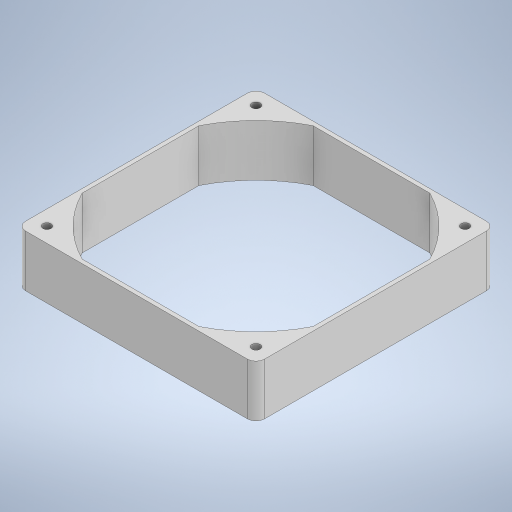
# Autodesk Inventor part: 120mm_fan
Saved by Autodesk Inventor 2023 (Build 270158000, 158)
## iProperties
Created: 2023-08-19
Part Number: 120mm_fan
Material: Generic
Document SubType Name: Modeling
Designer: plebbb
Density: 1 g/cm^3
Appearance: Default
Author: plebbb
Autodesk Inventor part; units mm, degrees
ref_plane "YZ Plane" through (0, 0, 0) normal (1, 0, 0) x (0, 1, 0)
ref_plane "XZ Plane" through (0, 0, 0) normal (0, 1, 0) x (-1, 0, 0)
ref_plane "XY Plane" through (0, 0, 0) normal (0, 0, 1) x (1, 0, 0)
sketch "Sketch1" plane through (0, 0, 0) normal (0, 1, 0) x (-1, 0, 0)
  line L0 (0, 0) -> (120, 0)
  line L1 (120, 0) -> (120, -120)
  line L2 (120, -120) -> (0, -120)
  line L3 (0, -120) -> (0, 0)
  line L4 (112.5, -7.5) -> (7.5, -7.5) construction
  line L5 (7.5, -7.5) -> (7.5, -112.5) construction
  line L6 (7.5, -112.5) -> (112.5, -112.5) construction
  line L7 (112.5, -112.5) -> (112.5, -7.5) construction
  line L8 (112.5, -60) -> (120, -60) construction
  line L9 (60, -112.5) -> (60, -120) construction
  circle A0 centre (112.5, -7.5) radius 2.1167
  circle A1 centre (112.5, -112.5) radius 2.1167
  circle A2 centre (7.5, -112.5) radius 2.1167
  circle A3 centre (7.5, -7.5) radius 2.1167
  circle A4 centre (60, -60) radius 65
  line L10 (89.3428, -2) -> (30.6572, -2)
  line L11 (118, -30.6572) -> (118, -89.3428)
  line L12 (89.3428, -118) -> (30.6572, -118)
  line L13 (2, -30.6572) -> (2, -89.3428)
  point P0 (116.25, -60)
  point P1 (60, -116.25)
  dimension "d3" = 130
  dimension "d0" = 120
  dimension "d1" = 105
  dimension "d2" = 4.2333
  dimension "d4" = 2
  constraints: 28 end point, 6 midpoint, 6 parallel, 5 equal length, 4 centre point, 4 perpendicular, 3 coincident, 3 equal radius, 3 horizontal, 1 horizontal alignment, 1 vertical, 1 vertical alignment, 10 other
  measures "d0" distance of L0.end L1.end
  measures "d1" distance of L6.end L4.start
  measures "d2" diameter of A0
  measures "d4" distance between parallel lines of L1 L11
extrude "Extrusion1" add sketch "Sketch1" along normal blind 26 contours L0 A4 L3 | L0 A4 L10 | A4 L13 L3 | L0 L1 A4 | A4 L2 L3 | L1 A4 L11 | A4 L12 L2 | L1 L2 A4
fillet "Fillet1" radius 4.2333 4 edges at (0, 13, -120) (-120, 13, -120) (-120, 13, 0) (0, 13, 0)
body "Solid1"
